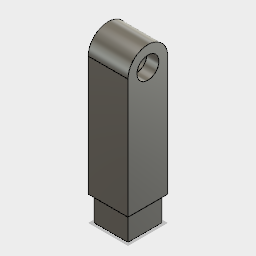
barras2 (Autodesk Fusion 360 design; units mm, degrees)
Autodesk Fusion 360 part; units mm, degrees
sketch "Sketch1" plane through (0, 0, 0) normal (0, 1, 0) x (1, 0, 0)
  line L0 (0, 17) -> (17, 17)
  line L1 (17, 17) -> (17, -17)
  line L2 (17, -17) -> (-17, -17)
  line L3 (-17, -17) -> (-17, 17)
  line L4 (-17, 17) -> (0, 17)
  dimension "d4" = 34
  dimension "d5" = 34
  measures "d4" distance of L1.end L2.end
  measures "d5" distance of L2.end L3.end
extrude "Extrude1" add sketch "Sketch1" along normal blind 25
sketch "Sketch2" plane through (0, 25, 0) normal (0, 1, 0) x (-1, 0, 0)
  line L0 (17, -17) -> (17, 17)
  line L1 (17, 17) -> (-17, 17)
  line L2 (-17, 17) -> (-17, -17)
  line L3 (-17, -17) -> (17, -17)
  line L4 (0, -20) -> (20, -20)
  line L5 (20, -20) -> (20, 20)
  line L6 (20, 20) -> (-20, 20)
  line L7 (-20, 20) -> (-20, -20)
  line L8 (-20, -20) -> (0, -20)
  dimension "d12" = 40
  measures "d12" distance of L6.end L7.end
extrude "Extrude2" add sketch "Sketch2" along normal blind 140 contours L0 L1 L2 L3 | L4 L5 L6 L7 L8
sketch "Sketch3" plane through (0, 165, 0) normal (0, 1, 0) x (-1, 0, 0)
  line L0 (-20, -20) -> (20, -20)
  line L1 (20, -20) -> (20, 20)
  line L2 (20, 20) -> (-20, 20)
  line L3 (-20, 20) -> (-20, -20)
  line L4 (0, -17) -> (17, -17)
  line L5 (17, -17) -> (17, 17)
  line L6 (17, 17) -> (-17, 17)
  line L7 (-17, 17) -> (-17, -17)
  line L8 (-17, -17) -> (0, -17)
  dimension "d19" = 34
  measures "d19" distance of L6.end L7.end
extrude "Extrude3" cut sketch "Sketch3" against normal blind 25 contours L4 L5 L6 L7 L8
extrude "Extrude4" add 1 faces at (5.6667, 140, -5.6667) along direction (0, 1, 0) blind 25
fillet "Fillet1" radius 20 2 edges at (0, 165, 20) (0, 165, -20)
hole "Hole1" at (20, 145, 0) direction (-1, 0, 0) diameter 22 depth 12 tip angle 118
